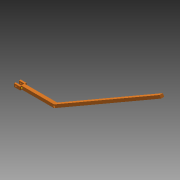
# Autodesk Inventor part: 3
Saved by Autodesk Inventor 2015 (Build 190159000, 159)
## iProperties
Created: 2016-03-16
Part Number: 3
Material: Złote
Document SubType Name: Modeling
Designer: Arek
Density: 19.3 g/cm^3
Appearance: Gorący metal 1600F
Mass: 23080.2 g
Surface Area: 1786.99 cm^2
Volume: 1195.87 cm^3
Author: Arek
Autodesk Inventor part; units mm, degrees
ref_plane "YZ Plane" through (0, 0, 0) normal (1, 0, 0) x (0, 1, 0)
ref_plane "XY Plane" through (0, 0, 0) normal (0, 0, 1) x (1, 0, 0)
sketch "Szkic1" plane through (0, 0, 0) normal (0, 1, 0) x (-1, 0, 0)
  line L0 (0, 15) -> (-300, 15)
  line L1 (-300, 15) -> (-300, -15)
  line L2 (-300, -15) -> (0, -15)
  line L3 (0, -15) -> (0, 15)
  line L4 (-300, 15) -> (-1278.6087, 580)
  line L5 (-1278.6087, 580) -> (-1291.5991, 557.5)
  line L6 (-300, -15) -> (-1291.5991, 557.5)
  point P0 (0, 0)
  point P1 (0, 0)
  dimension "d0" = 300
  dimension "d1" = 30
  dimension "d2" = 150
  dimension "d3" = 1130
  constraints: 14 end point, 3 parallel, 2 coincident, 2 perpendicular, 1 horizontal, 1 midpoint
  measures "d0" distance of L2.end L1.end
  measures "d1" distance of L1.end L0.end
  measures "d2" angle of L4 L0
  measures "d3" distance of L0.end L4.end
extrude "Wyciągnięcie proste1" add sketch "Szkic1" along normal blind 30
sketch "Szkic2" plane through (0, 30, 0) normal (0, 1, 0) x (1, 0, 0)
  circle A0 centre (300, 0) radius 10
  line L0 (300, 15) -> (0, 15) projected
  point P0 (0, 0)
  dimension "d6" = 20
  dimension "d7" = 15
  constraints: 1 centre point, 1 vertical alignment
  measures "d6" diameter of A0
  measures "d7" distance from line of L0 A0.centre
extrude "Wyciągnięcie proste2" cut sketch "Szkic2" against normal through all
sketch "Szkic3" plane through (0, 0, -15) normal (-1, 0, 0) x (0, 0, 1)
  point P0 (15, 0)
sketch "Szkic4" plane through (0, 0, -15) normal (-1, 0, 0) x (0, 0, 1)
  line L0 (0, 0) -> (30, 0) projected
  line L1 (30, 0) -> (30, 30) projected
  line L2 (0, 30) -> (30, 30) projected
  line L3 (0, 0) -> (0, 30) projected
  line L4 (30, 45) -> (0, 45)
  line L5 (0, 45) -> (0, -15)
  line L6 (0, -15) -> (30, -15)
  line L7 (30, -15) -> (30, 45)
  line L8 (30, 45) -> (0, -15) construction
  line L9 (0, 45) -> (30, -15) construction
  point P0 (15, 0)
  point P1 (15, 15)
  dimension "d10" = 30
  dimension "d11" = 60
  dimension "d12" = 0
  dimension "d13" = 15
  constraints: 12 end point, 2 midpoint, 2 parallel, 1 horizontal, 1 perpendicular
  measures "d10" distance of L6.end L5.end
  measures "d11" distance of L5.end L4.end
  measures "d12" distance between parallel lines of L1 L7
  measures "d13" distance between parallel lines of L2 L4
extrude "Wyciągnięcie proste3" add sketch "Szkic4" along normal blind 5
sketch "Szkic5" plane through (-5, 0, -15) normal (-1, 0, 0) x (0, 0, 1)
  line L0 (0, -15) -> (30, -15)
  line L1 (30, -15) -> (30, 0)
  line L2 (30, 0) -> (0, 0)
  line L3 (0, 0) -> (0, -15)
  point P0 (15, 0)
  dimension "d16" = 30
  dimension "d17" = 15
  constraints: 8 end point, 2 parallel, 1 horizontal, 1 perpendicular
  measures "d16" distance of L2.end L1.end
  measures "d17" distance of L1.end L0.end
extrude "Wyciągnięcie proste4" add sketch "Szkic5" along normal blind 50
ref_plane "Płaszczyzna konstrukcyjna1" through (0, 15, 0) normal (0, 1, 0) x (-1, 0, 0)
mirror "Odbicie lustrzane1" about plane through (0, 15, 0) normal (0, 1, 0) of "Wyciągnięcie proste4"
sketch "Szkic6" plane through (0, 45, 15) normal (0, 1, 0) x (1, 0, 0)
  circle A0 centre (-40, 15) radius 7.5
  line L0 (-55, 30) -> (-55, 0) projected
  line L1 (0, 0) -> (0, 30) projected
  point P0 (0, 15)
  point P1 (0, 15)
  dimension "d21" = 15
  dimension "d22" = 15
  constraints: 1 centre point, 1 horizontal alignment, 1 midpoint
  measures "d21" diameter of A0
  measures "d22" distance from line of L0 A0.centre
extrude "Wyciągnięcie proste5" cut sketch "Szkic6" against normal through all
